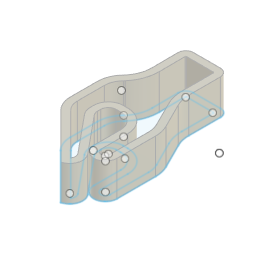
Chip Clip Hand v1 (Autodesk Fusion 360 design; units mm, degrees)
Autodesk Fusion 360 part; units mm, degrees
sketch "Sketch1" plane through (0, 0, 0) normal (0, 0, 1) x (1, 0, 0)
  line L0 (3.309, 32.844) -> (14.9188, 32.844)
  line L1 (26.2752, -6.3858) -> (26.2752, -22.9908)
  arc A0 (16.422, -22.9908) -> (26.2752, -22.9908) centre (21.3486, -22.9908) ccw
  line L2 (16.422, -22.9908) -> (16.422, -11.4954)
  line L3 (5.3015, -11.7323) -> (18.4305, -27.6914)
  arc A1 (15.6271, -36.4434) -> (18.4305, -27.6914) centre (14.2091, -31.1642) ccw
  line L4 (15.6271, -36.4434) -> (-3.6897, -17.1266)
  line L5 (-6.5756, -10.1593) -> (-6.5756, 1.4585)
  line L6 (-3.2683, 9.443) -> (-3.7397, 8.9716)
  line L7 (0.1079, 18.3592) -> (0.0246, 29.5352)
  line L8 (18.2032, 29.5596) -> (18.2032, 15.961)
  line L9 (19.5902, 10.0856) -> (24.8883, -0.5105)
  arc A2 (-3.2683, 9.443) -> (-6.5756, 1.4585) centre (4.7161, 1.4585) ccw
  line L10 (9.8532, -4.9266) -> (7.8379, -4.9266)
  line L11 (4.5535, -8.211) -> (4.5535, -9.6457)
  arc A3 (7.8379, -4.9266) -> (4.5535, -8.211) centre (7.8379, -8.211) ccw
  arc A4 (4.5535, -9.6457) -> (5.3015, -11.7323) centre (7.8379, -9.6457) ccw
  arc A5 (16.422, -11.4954) -> (9.8532, -4.9266) centre (9.8532, -11.4954) ccw
  arc A6 (-6.5756, -10.1593) -> (-3.6897, -17.1266) centre (3.2776, -10.1593) ccw
  arc A7 (26.2752, -6.3858) -> (24.8883, -0.5105) centre (13.1376, -6.3858) ccw
  arc A8 (18.2032, 15.961) -> (19.5902, 10.0856) centre (31.3409, 15.961) ccw
  arc A9 (-3.7397, 8.9716) -> (0.1079, 18.3592) centre (-13.0294, 18.2613) ccw
  arc A10 (3.309, 32.844) -> (0.0246, 29.5352) centre (3.309, 29.5596) ccw
  arc A11 (18.2032, 29.5596) -> (14.9188, 32.844) centre (14.9188, 29.5596) ccw
  arc A12 (-1.147, 7.3217) -> (-3.5756, 1.4585) centre (4.7161, 1.4585) ccw
  line L12 (-3.5756, -10.1593) -> (-3.5756, 1.4585)
  arc A13 (-3.5756, -10.1593) -> (-1.5683, -15.0053) centre (3.2776, -10.1593) ccw
  line L13 (16.1333, -32.7069) -> (-1.5683, -15.0053)
  arc A14 (16.1333, -32.7069) -> (16.1137, -29.5973) centre (14.2091, -31.1642) ccw
  line L14 (2.9847, -13.6383) -> (16.1137, -29.5973)
  arc A15 (1.5535, -9.6457) -> (2.9847, -13.6383) centre (7.8379, -9.6457) ccw
  line L15 (1.5535, -8.211) -> (1.5535, -9.6457)
  arc A16 (7.8379, -1.9266) -> (1.5535, -8.211) centre (7.8379, -8.211) ccw
  line L16 (9.8532, -1.9266) -> (7.8379, -1.9266)
  arc A17 (19.422, -11.4954) -> (9.8532, -1.9266) centre (9.8532, -11.4954) ccw
  line L17 (19.422, -22.9908) -> (19.422, -11.4954)
  arc A18 (19.422, -22.9908) -> (23.2752, -22.9908) centre (21.3486, -22.9908) ccw
  line L18 (23.2752, -6.3858) -> (23.2752, -22.9908)
  arc A19 (23.2752, -6.3858) -> (22.205, -1.8521) centre (13.1376, -6.3858) ccw
  line L19 (16.9069, 8.744) -> (22.205, -1.8521)
  arc A20 (15.2032, 15.961) -> (16.9069, 8.744) centre (31.3409, 15.961) ccw
  line L20 (15.2032, 29.5596) -> (15.2032, 15.961)
  arc A21 (15.2032, 29.5596) -> (14.9188, 29.844) centre (14.9188, 29.5596) ccw
  line L21 (3.309, 29.844) -> (14.9188, 29.844)
  arc A22 (3.309, 29.844) -> (3.0246, 29.5575) centre (3.309, 29.5596) ccw
  line L22 (3.1078, 18.3815) -> (3.0246, 29.5575)
  arc A23 (-0.8215, 7.7071) -> (3.1078, 18.3815) centre (-13.0294, 18.2613) ccw
  arc A24 (-1.147, 7.3217) -> (-0.8215, 7.7071) centre (-3.2683, 9.443) ccw
  dimension "d13" = 3
  constraint horizontal L0
  constraint perpendicular L0 L1
  constraint tangent L1 A0
  constraint tangent A0 L2
  constraint perpendicular L0 L2
  constraint tangent L3 A1
  constraint vertical L5
  constraint perpendicular L4 L6
  constraint perpendicular L0 L8
  constraint tangent L6 A2
  constraint tangent L5 A2
  constraint horizontal L10
  constraint perpendicular L10 L11
  constraint tangent L10 A3
  constraint tangent L11 A3
  constraint tangent L3 A4
  constraint tangent L11 A4
  constraint equal A3 A4
  constraint tangent L10 A5
  constraint tangent L2 A5
  constraint tangent L5 A6
  constraint tangent L4 A6
  constraint tangent L9 A7
  constraint tangent L1 A7
  constraint tangent L8 A8
  constraint tangent L9 A8
  constraint equal A7 A8
  constraint tangent L6 A9
  constraint tangent L7 A9
  constraint equal A7 A9
  constraint tangent L0 A10
  constraint tangent L7 A10
  constraint tangent L8 A11
  constraint tangent L0 A11
extrude "Extrude1" add sketch "Sketch1" along normal blind 15
sketch "Sketch2" plane through (0, 0, 0) normal (0, 1, 0) x (1, 0, 0)
